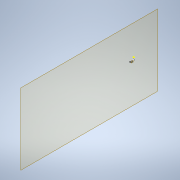
# Autodesk Inventor part: topwaterpipes
Saved by Autodesk Inventor 2020 (Build 240168000, 168)
## iProperties
Created: 2019-07-31
Part Number: topwaterpipes
Material: Generic
Document SubType Name: Modeling
Designer: ColinP
Density: 1 g/cm^3
Appearance: Default
Author: ColinP
Autodesk Inventor part; units mm, degrees
ref_plane "YZ Plane" through (0, 0, 0) normal (1, 0, 0) x (0, 1, 0)
ref_plane "XZ Plane" through (0, 0, 0) normal (0, 1, 0) x (-1, 0, 0)
ref_plane "XY Plane" through (0, 0, 0) normal (0, 0, 1) x (1, 0, 0)
sketch "Sketch1" plane through (0, 0, 0) normal (0, 0, 1) x (1, 0, 0)
  circle A0 centre (3.175, -9.6512) radius 3.175 projected
  circle A1 centre (3.175, 9.6512) radius 3.175 projected
  circle A2 centre (3.175, -9.6512) radius 3.048
  point P0 (0, 0)
  dimension "d0" = 6.096
  constraints: 1 centre point, 1 coincident
  measures "d0" diameter of A2
extrude "Extrusion1" add sketch "Sketch1" along normal blind 16.51 contours A0
ref_plane "Work Plane1" through (0, 0, 298.4246) normal (1, 0, 0) x (0, 0, 1)
sketch "Sketch2" plane through (0, 0, 298.4246) normal (1, 0, 0) x (0, 0, 1)
  point P0 (-298.4246, 0)
ref_plane "Work Plane2" through (6.985, -9.6512, 9.8182) normal (-1, 0, 0) x (0, 0, 1)
sketch "Sketch3" plane through (6.985, -9.6512, 9.8182) normal (-1, 0, 0) x (0, 0, 1)
  circle A0 centre (1.5875, 0) radius 3.175 projected
  circle A1 centre (1.5875, 0) radius 1.143 projected
  point P0 (-9.8182, 9.6512)
extrude "Extrusion2" cut sketch "Sketch3" along normal blind 3.81 contours A0 | A1
sketch "Sketch4" plane through (3.175, -9.6512, 9.8182) normal (1, 0, 0) x (0, 0, -1)
  arc A0 (-1.5875, 3.175) -> (-1.5875, -3.175) centre (-1.5875, 0) ccw projected
  circle A1 centre (-1.5875, 0) radius 3.175
  circle A2 centre (-1.5875, 0) radius 3.048
  point P0 (9.8182, 9.6512)
  dimension "d6" = 6.35
  dimension "d7" = 6.096
  constraints: 2 centre point, 2 coincident
  measures "d6" diameter of A1
  measures "d7" diameter of A2
extrude "Extrusion3" add sketch "Sketch4" along normal blind 3.81
sketch "Sketch5" plane through (3.175, -9.6512, 9.8182) normal (-1, 0, 0) x (0, 0, 1)
  point P0 (-9.8182, 9.6512)
sketch "Sketch6" plane through (3.175, -9.6512, 16.51) normal (0, 0, 1) x (1, 0, 0)
  circle A0 centre (0, 0) radius 3.048 projected
  circle A1 centre (0, 0) radius 3.175 projected
  point P0 (-3.175, 9.6512)
extrude "Extrusion4" cut sketch "Sketch6" against normal through all contours A0
extrude "Extrusion5" add sketch "Sketch6" along normal blind 1.27 contours A0 | A1
body "Solid1"
